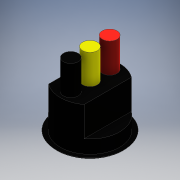
# Autodesk Inventor part: Switch_DC_Pilot
Saved by Autodesk Inventor 2016 (Build 200138000, 138)
## iProperties
Created: 2019-09-20
Part Number: Switch_DC_Pilot
Material: Generic
Document SubType Name: Modeling
Designer: jimmy
Density: 1 g/cm^3
Appearance: Default
Author: jimmy
Autodesk Inventor part; units mm, degrees
ref_plane "YZ Plane" through (0, 0, 0) normal (1, 0, 0) x (0, 1, 0)
ref_plane "XZ Plane" through (0, 0, 0) normal (0, 1, 0) x (-1, 0, 0)
ref_plane "XY Plane" through (0, 0, 0) normal (0, 0, 1) x (1, 0, 0)
sketch "Sketch1" plane through (0, 0, 0) normal (0, 0, 1) x (1, 0, 0)
  circle A0 centre (0, 0) radius 10
  dimension "d0" = 20
  constraints: 1 centre point, 1 coincident
  measures "d0" diameter of A0
extrude "Extrusion1" add sketch "Sketch1" along normal blind 4.5
sketch "Sketch2" plane through (0, 0, 4.5) normal (0, 0, 1) x (1, 0, 0)
  circle A0 centre (0, 0) radius 10 projected
  line L0 (-6, -8) -> (6, -8)
  line L1 (6, -8) -> (6, 8)
  line L2 (6, 8) -> (-6, 8)
  line L3 (-6, 8) -> (-6, -8)
  line L4 (-6, -8) -> (6, 8) construction
  line L5 (6, -8) -> (-6, 8) construction
  arc A1 (6, 8) -> (-6, 8) centre (0, 0) ccw
  arc A2 (-6, -8) -> (6, -8) centre (0, 0) ccw
  dimension "d3" = 12
  constraints: 12 end point, 4 point on circle, 2 centre point, 2 midpoint, 2 parallel, 1 horizontal, 1 perpendicular, 2 other
  measures "d3" distance of L2.end L1.end
extrude "Extrusion2" add sketch "Sketch2" along normal blind 10 contours L2 A0 | L1 L0 L3 L2 | A0 L0
sketch "Sketch3" plane through (0, 0, 0) normal (0, 0, -1) x (-1, 0, 0)
  circle A0 centre (0, 0) radius 11.5
  dimension "d6" = 23
  constraints: 1 centre point, 1 coincident
  measures "d6" diameter of A0
extrude "Extrusion3" add sketch "Sketch3" along normal blind 1
fillet "Fillet1" radius 2 1 edges at (11.5, 0, -1)
sketch "Sketch4" plane through (0, 0, 14.5) normal (0, 0, 1) x (1, 0, 0)
  circle A0 centre (0, 6.6483) radius 2.5
  circle A1 centre (0, 0) radius 2.5
  circle A2 centre (0, -6.4728) radius 2.5
  dimension "d10" = 5
  dimension "d11" = 5
  dimension "d12" = 5
  constraints: 3 centre point, 1 coincident
  measures "d10" diameter of A0
  measures "d11" diameter of A1
  measures "d12" diameter of A2
extrude "Extrusion4" add sketch "Sketch4" along normal blind 10
body "Solid1"
